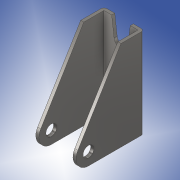
# Autodesk Inventor part: Mount
Saved by Autodesk Inventor 2017 SP1 (Build 210196100, 196)
## iProperties
Created: 2017-08-20
Part Number: Mount
Material: Stainless Steel
Document SubType Name: Modeling
Designer: Zach
Density: 8 g/cm^3
Appearance: Semi-Polished
Author: Zach
Autodesk Inventor part; units mm, degrees
ref_plane "YZ Plane" through (0, 0, 0) normal (1, 0, 0) x (0, 1, 0)
ref_plane "XZ Plane" through (0, 0, 0) normal (0, 1, 0) x (-1, 0, 0)
ref_plane "XY Plane" through (0, 0, 0) normal (0, 0, 1) x (1, 0, 0)
sketch "Sketch1" plane through (0, 0, 0) normal (0, 0, 1) x (1, 0, 0)
  line L0 (0, 0) -> (26, 0)
  line L1 (26, 0) -> (26, 58)
  line L2 (26, 58) -> (0, 58) construction
  line L3 (0, 58) -> (0, 0)
  circle A0 centre (13, 16) radius 3
  line L4 (0, 58) -> (7, 58)
  line L5 (19, 58) -> (26, 58)
  line L6 (17.464, 45.9318) -> (19, 58)
  line L7 (8.536, 45.9318) -> (7, 58)
  line L8 (13, 58) -> (13, 46.5) construction
  circle A1 centre (13, 46.5) radius 4.5 construction
  arc A2 (8.536, 45.9318) -> (17.464, 45.9318) centre (13, 46.5) ccw
  point P0 (13, 0)
  dimension "d0" = 26
  dimension "d1" = 58
  dimension "d2" = 6
  dimension "d3" = 16
  dimension "d19" = 12
  dimension "d20" = 9
  dimension "d21" = 11.5
  constraints: 20 end point, 4 point on circle, 3 centre point, 2 collinear, 2 midpoint, 2 parallel, 2 point on line, 1 coincident, 1 concentric, 1 horizontal, 1 perpendicular, 1 tangent, 1 vertical, 1 vertical alignment, 1 other
  measures "d0" distance of L2.end L1.end
  measures "d1" distance of L1.end L0.end
  measures "d2" diameter of A0
  measures "d3" distance from line of L0 A0.centre
  measures "d19" distance of L4.end L5.start
  measures "d20" diameter of A1
  measures "d21" distance of L8.start L8.end
extrude "Extrusion1" add sketch "Sketch1" along normal blind 2
sketch "Sketch2" plane through (26, 0, 0) normal (1, 0, 0) x (0, 0, -1)
  circle A0 centre (-36, 8) radius 3.5
  line L0 (0, 0) -> (0, 58) projected
  line L1 (0, 0) -> (-36, 0)
  circle A1 centre (-36, 8) radius 8 construction
  line L2 (0, 58) -> (-15, 58)
  line L3 (-15, 58) -> (-42.8382, 12.152)
  arc A2 (-42.8382, 12.152) -> (-36, 0) centre (-36, 8) ccw
  dimension "d13" = 16
  dimension "d8" = 7
  dimension "d10" = 8
  dimension "d11" = 36
  dimension "d14" = 15
  constraints: 6 end point, 2 centre point, 2 horizontal, 2 point on circle, 1 coincident, 6 other
  measures "d8" diameter of A0
  measures "d10" vertical distance of L0.start A0.centre
  measures "d11" distance from line of L0 A0.centre
  measures "d14" distance of L0.end L2.end
extrude "Extrusion2" add sketch "Sketch2" against normal blind 2
sketch "Sketch3" plane through (0, 0, 0) normal (-1, 0, 0) x (0, 0, 1)
  line L0 (2, 0) -> (2, 58) projected
  line L1 (2, 0) -> (36, 0) projected
  arc A0 (36, 0) -> (42.8382, 12.152) centre (36, 8) ccw projected
  line L2 (42.8382, 12.152) -> (15, 58) projected
  line L3 (15, 58) -> (2, 58) projected
  circle A1 centre (36, 8) radius 3.5 projected
  point P0 (0, 0)
extrude "Extrusion3" add sketch "Sketch3" against normal blind 2
fillet "Fillet1" radius 2 2 edges at (0, 29, 0) (26, 29, 0)
body "Solid1"
